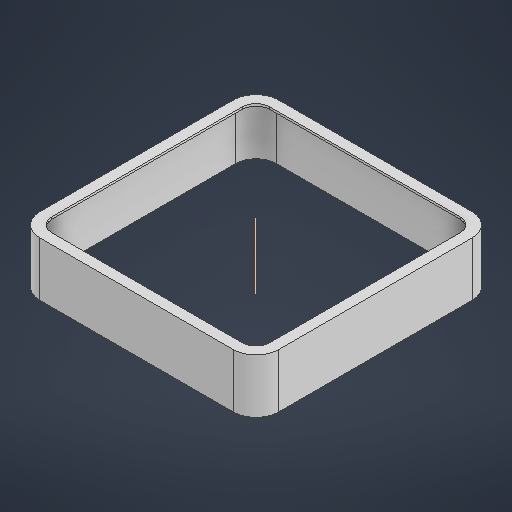
# Autodesk Inventor part: m5stack_cover
Saved by Autodesk Inventor 2026 (Build 300175000, 175)
## iProperties
Created: 2025-05-07
Part Number: m5stack_cover
Material: Generic
Document SubType Name: Modeling
Designer: Paul Juschitz
Density: 1 g/cm^3
Appearance: Default
Author: Paul Juschitz
Autodesk Inventor part; units mm, degrees
ref_plane "YZ Plane" through (0, 0, 0) normal (1, 0, 0) x (0, 1, 0)
ref_plane "XZ Plane" through (0, 0, 0) normal (0, 1, 0) x (-1, 0, 0)
ref_plane "XY Plane" through (0, 0, 0) normal (0, 0, 1) x (1, 0, 0)
sketch "Sketch1" plane through (0, 0, 0) normal (0, 1, 0) x (-1, 0, 0)
  line L0 (25.2, -25.2) -> (-25.2, -25.2) construction
  line L1 (-25.2, -25.2) -> (-25.2, 25.2) construction
  line L2 (-25.2, 25.2) -> (25.2, 25.2) construction
  line L3 (25.2, 25.2) -> (25.2, -25.2) construction
  line L4 (25.2, -25.2) -> (-25.2, 25.2) construction
  line L5 (-25.2, -25.2) -> (25.2, 25.2) construction
  arc A0 (22, -25.2) -> (25.2, -22) centre (22, -22) ccw
  arc A1 (-25.2, -22) -> (-22, -25.2) centre (-22, -22) ccw
  arc A2 (25.2, 22) -> (22, 25.2) centre (22, 22) ccw
  arc A3 (-22, 25.2) -> (-25.2, 22) centre (-22, 22) ccw
  line L6 (22, -25.2) -> (-22, -25.2)
  line L7 (-25.2, -22) -> (-25.2, 22)
  line L8 (-22, 25.2) -> (22, 25.2)
  line L9 (25.2, 22) -> (25.2, -22)
  line L10 (0, -60) -> (0, 60) construction
  line L11 (60, 0) -> (-60, 0) construction
  line L12 (27.6, -22.3674) -> (27.6, 22.3674)
  arc A4 (27.6, 22.3674) -> (22.3674, 27.6) centre (22.3674, 22.3674) ccw
  line L13 (22.3674, 27.6) -> (-22.3674, 27.6)
  arc A5 (-22.3674, 27.6) -> (-27.6, 22.3674) centre (-22.3674, 22.3674) ccw
  line L14 (-27.6, 22.3674) -> (-27.6, -22.3674)
  arc A6 (-27.6, -22.3674) -> (-22.3674, -27.6) centre (-22.3674, -22.3674) ccw
  line L15 (-22.3674, -27.6) -> (22.3674, -27.6)
  arc A7 (22.3674, -27.6) -> (27.6, -22.3674) centre (22.3674, -22.3674) ccw
  point P0 (0, 0)
  point P1 (26.0674, -26.0674)
  dimension "d0" = 50.4
  dimension "d1" = 6.4
  dimension "d2" = 120
  dimension "d3" = 120
  dimension "d4" = 55.2
  dimension "d5" = 3.7
  constraints: 32 end point, 17 point on circle, 12 point on line, 12 tangent, 8 centre point, 6 equal radius, 6 perpendicular, 4 midpoint, 3 vertical, 2 parallel, 1 horizontal, 2 other
  measures "d0" distance of L1.end L2.end
  measures "d1" diameter of A0
  measures "d2" distance of L10.start L10.end
  measures "d3" distance of L11.start L11.end
  measures "d4" distance between parallel lines of L14 L12
  measures "d5" horizontal distance of point (26.067, -26.067) A7.centre
extrude "Extrusion1" add sketch "Sketch1" against normal blind 0.5
sketch "Sketch2" plane through (0, -0.5, 0) normal (0, -1, 0) x (1, 0, 0)
  line L0 (-27.6, 22.3674) -> (-27.6, -22.3674) projected
  arc A0 (-22.3674, 27.6) -> (-27.6, 22.3674) centre (-22.3674, 22.3674) ccw projected
  line L1 (22.3674, 27.6) -> (-22.3674, 27.6) projected
  arc A1 (27.6, 22.3674) -> (22.3674, 27.6) centre (22.3674, 22.3674) ccw projected
  line L2 (27.6, -22.3674) -> (27.6, 22.3674) projected
  arc A2 (22.3674, -27.6) -> (27.6, -22.3674) centre (22.3674, -22.3674) ccw projected
  line L3 (-22.3674, -27.6) -> (22.3674, -27.6) projected
  arc A3 (-27.6, -22.3674) -> (-22.3674, -27.6) centre (-22.3674, -22.3674) ccw projected
  line L4 (-27.1, 22.3674) -> (-27.1, -22.3674)
  arc A4 (-27.1, -22.3674) -> (-22.3674, -27.1) centre (-22.3674, -22.3674) ccw
  line L5 (-22.3674, -27.1) -> (22.3674, -27.1)
  arc A5 (22.3674, -27.1) -> (27.1, -22.3674) centre (22.3674, -22.3674) ccw
  line L6 (27.1, -22.3674) -> (27.1, 22.3674)
  arc A6 (27.1, 22.3674) -> (22.3674, 27.1) centre (22.3674, 22.3674) ccw
  line L7 (22.3674, 27.1) -> (-22.3674, 27.1)
  arc A7 (-22.3674, 27.1) -> (-27.1, 22.3674) centre (-22.3674, 22.3674) ccw
  point P0 (0, 0)
  dimension "d8" = 0.5
  constraints: 8 end point, 8 point on circle, 4 centre point, 7 other
  measures "d8" radial gap between concentric circles of A0 A7
extrude "Extrusion2" add sketch "Sketch2" along normal blind 12
equation "\"d0\" = m5stack_inner_width"
equation "\"d1\" = 2 * m5stack_inner_coner_radius"
equation "\"d4\" = m5stack_outer_width + 2 * casing_tolerance + 2 * casing_thickness"
equation "\"d5\" = 0.5 * m5stack_outer_corner_radius + 2 * casing_tolerance + 2 * casing_thickness"
equation "\"d6\" = casing_thickness"
equation "\"d8\" = casing_thickness"
equation "\"m5stack_outer_width\" = 54"
equation "\"m5stack_outer_corner_radius\" = 5"
equation "\"m5stack_inner_width\" = 50.4"
equation "\"m5stack_inner_coner_radius\" = 3.2"
equation "\"casing_tolerance\" = 0.1"
equation "\"casing_thickness\" = 0.5"
body "Solid1"
